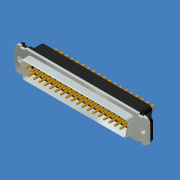
# Autodesk Inventor part: DBConnector
Saved by Autodesk Inventor 2019 (Build 230136000, 136)
## iProperties
Shininess: 64.0
Angle Display Precision: 2
Document Length Units: 11272
Document Angle Units: 11279
Document Time Units: 11290
Document Mass Units: 11286
Document Length Units Precision: 3
Document Angle Units Precision: 2
Compacted: True
Created: 2001-12-01
Part Number: DBConnector
Description: Dsub 37 Pin, 2 Row, Male
Document SubType Name: Modeling
Designer: Charles Bliss
Material: Generic
Density: 1 g/cm^3
Appearance: Zinc
Categories: <MemberInstance><Categories><Category DisplayName="" Mnemonic="CABLEANDHARNESS" InternalName="e4a7e005-5e42-4d16-b293-125e7f0d0512"><Category DisplayName="" Mnemonic="CONNECTORS" InternalName="6f634eba-a678-4820-a31d-2c2d5ee6728e"><CategoryParameter DisplayName="" Mnemonic="REFDES" InternalName="c3740e8c-60ab-4d5d-8584-52b73222f2f0"/><Category DisplayName="" Mnemonic="RIBBONCABLE" InternalName="27621a3d-53ec-49ed-8225-e2ac65e8eb52"/></Category></Category></Categories><FamilyTemplate><FamilyTemplateParameters></FamilyTemplateParameters></FamilyTemplate><CategoryParameterMap><ParamToTemplateMap><ParamToTemplate CategoryParameter="//CategoryParameter[@InternalName='c3740e8c-60ab-4d5d-8584-52b73222f2f0']" ConstantValue=""/></ParamToTemplateMap></CategoryParameterMap></MemberInstance>
Density: 0.0
Volumn: 0.0
Area: 0.0
PropertySet Name: Model Information
Control State: 0
Master: False
Checked Out: False
Author: Charles Bliss
Autodesk Inventor part; units mm, degrees
ref_plane "YZ Plane" through (0, 0, 0) normal (1, 0, 0) x (0, 1, 0)
ref_plane "XZ Plane" through (0, 0, 0) normal (0, 1, 0) x (-1, 0, 0)
ref_plane "XY Plane" through (0, 0, 0) normal (0, 0, 1) x (1, 0, 0)
sketch "Sketch1" plane through (0, 0, 0) normal (0, 0, 1) x (1, 0, 0)
  line L0 (-29.3316, 6.2738) -> (29.3316, 6.2738)
  line L1 (29.3316, 6.2738) -> (29.3316, 5.4179)
  line L2 (29.3316, 5.4179) -> (31.75, 5.4179)
  line L3 (31.75, 5.4179) -> (31.75, 6.2738)
  line L4 (31.75, 6.2738) -> (32.2399, 6.2738)
  arc A0 (34.6583, 3.8554) -> (32.2399, 6.2738) centre (32.2399, 3.8554) ccw
  line L5 (-29.3316, 6.2738) -> (-29.3316, 5.4179)
  line L6 (-29.3316, 5.4179) -> (-31.75, 5.4179)
  line L7 (-31.75, 5.4179) -> (-31.75, 6.2738)
  line L8 (-31.75, 6.2738) -> (-32.2399, 6.2738)
  arc A1 (-32.2399, 6.2738) -> (-34.6583, 3.8554) centre (-32.2399, 3.8554) ccw
  line L9 (-34.6583, 0) -> (34.6583, 0) construction
  line L10 (-29.3316, -6.2738) -> (29.3316, -6.2738)
  line L11 (-29.3316, -6.2738) -> (-29.3316, -5.4179)
  line L12 (-29.3316, -5.4179) -> (-31.75, -5.4179)
  line L13 (-31.75, -5.4179) -> (-31.75, -6.2738)
  line L14 (-31.75, -6.2738) -> (-32.2399, -6.2738)
  arc A2 (-34.6583, -3.8554) -> (-32.2399, -6.2738) centre (-32.2399, -3.8554) ccw
  line L15 (29.3316, -6.2738) -> (29.3316, -5.4179)
  line L16 (29.3316, -5.4179) -> (31.75, -5.4179)
  line L17 (31.75, -5.4179) -> (31.75, -6.2738)
  line L18 (31.75, -6.2738) -> (32.2399, -6.2738)
  arc A3 (32.2399, -6.2738) -> (34.6583, -3.8554) centre (32.2399, -3.8554) ccw
  line L19 (-34.6583, 3.8554) -> (-34.6583, -3.8554)
  line L20 (34.6583, 3.8554) -> (34.6583, -3.8554)
  line L21 (-27.1708, -3.1583) -> (-28.0576, 1.8711)
  arc A4 (-25.802, 4.5593) -> (-28.0576, 1.8711) centre (-25.802, 2.2689) ccw
  line L22 (-25.802, 4.5593) -> (25.802, 4.5593)
  arc A5 (28.0576, 1.8711) -> (25.802, 4.5593) centre (25.802, 2.2689) ccw
  line L23 (28.0576, 1.8711) -> (27.1708, -3.1583)
  arc A6 (25.5011, -4.5593) -> (27.1708, -3.1583) centre (25.5011, -2.8639) ccw
  line L24 (25.5011, -4.5593) -> (-25.5011, -4.5593)
  arc A7 (-27.1708, -3.1583) -> (-25.5011, -4.5593) centre (-25.5011, -2.8639) ccw
  line L25 (0, 6.2738) -> (0, -6.2738) construction
  line L26 (0, 4.5593) -> (0, -4.5593) construction
  line L27 (-25.5011, -4.1783) -> (25.5011, -4.1783)
  arc A8 (25.5011, -4.1783) -> (26.7956, -3.0921) centre (25.5011, -2.8639) ccw
  line L28 (26.7956, -3.0921) -> (27.6824, 1.9373)
  arc A9 (27.6824, 1.9373) -> (25.802, 4.1783) centre (25.802, 2.2689) ccw
  line L29 (25.802, 4.1783) -> (-25.802, 4.1783)
  arc A10 (-25.802, 4.1783) -> (-27.6824, 1.9373) centre (-25.802, 2.2689) ccw
  line L30 (-27.6824, 1.9373) -> (-26.7956, -3.0921)
  arc A11 (-26.7956, -3.0921) -> (-25.5011, -4.1783) centre (-25.5011, -2.8639) ccw
  circle A12 centre (-31.75, 0) radius 1.524
  circle A13 centre (31.75, 0) radius 1.524
  line L31 (-31.75, 0) -> (0, 0) construction
  line L32 (0, 0) -> (31.75, 0) construction
  line L33 (27.7114, 6.2738) -> (27.7114, 2.2689) construction
  line L34 (-27.7114, 6.2738) -> (-27.7114, 2.2689) construction
  line L35 (-27.9785, 1.4224) -> (27.9785, 1.4224) construction
  line L36 (-27.4769, -1.4224) -> (27.4769, -1.4224) construction
  circle A14 centre (-25.146, 1.4224) radius 0.4953
  circle A15 centre (-23.749, -1.4224) radius 0.4953
  line L37 (-26.9753, -4.2672) -> (26.9753, -4.2672) construction
  circle A16 centre (-25.146, -4.2672) radius 0.4953
  point P0 (0, -1.4224)
  dimension "d0" = 10
  dimension "HoleCtr" = 63.5
  dimension "OAL" = 69.3166
  dimension "ShellLen" = 55.4228
  dimension "ShellWid" = 8.3566
  dimension "HoleDia" = 3.048
  dimension "d6" = 0.381
  dimension "d7" = 2.4184
  dimension "d8" = 0.8559
  dimension "d9" = 2.4184
  dimension "OAW" = 12.5476
  dimension "d11" = 1.3144
  dimension "PinVertDist" = 2.8448
  dimension "PinDia" = 0.9906
  dimension "Pin1Offset" = 25.146
  dimension "d19" = 1.397
  dimension "d34" = 1.9094
  dimension "CLoffset" = 2.7559
  dimension "d52" = 2.8448
  constraints: 76 end point, 26 point on circle, 17 centre point, 16 tangent, 14 point on line, 14 symmetric about line, 10 parallel, 8 midpoint, 6 equal length, 6 equal radius, 5 collinear, 4 perpendicular, 3 horizontal, 3 vertical alignment, 2 coincident, 2 vertical, 18 other
  measures "d0" angle of L21 L19
  measures "HoleCtr" diameter of A12.centre L25
  measures "OAL" distance between parallel lines of L20 L19
  measures "ShellLen" distance between parallel lines of L33 L34
  measures "ShellWid" distance between parallel lines of L27 L29
  measures "HoleDia" diameter of A13
  measures "d6" distance between parallel lines of L30 L21
  measures "d7" distance of L6.start L6.end
  measures "d8" distance of L0.start L6.start
  measures "d9" radius of A1
  measures "OAW" distance between parallel lines of L10 L0
  measures "d11" radius of A8
  measures "PinVertDist" distance between parallel lines of L36 L35
  measures "PinDia" diameter of A15
  measures "Pin1Offset" distance from line of A14.centre L26
  measures "d19" horizontal distance of A15.centre A14.centre
  measures "d34" radius of A10
  measures "CLoffset" distance between parallel lines of L27 L36
  measures "d52" distance between parallel lines of L37 L36
extrude "Extrusion1" add sketch "Sketch1" along normal blind 1.27 contours L0 L1 L2 L3 L4 A0 L20 A3 L18 L17 L16 L15 L10 L11 L12 L13 L14 A2 L19 A1 L8 L7 L6 L5 | L21 A4 L22 A5 L23 A6 L24 A16 L27 A8 L28 A9 L29 A10 L30 A11 A7 | A16 A11 L27 L24 A7 | A7 L24 A16
extrude "Extrusion2" add sketch "Sketch1" along normal blind 5.08 contours L21 A4 L22 A5 L23 A6 L24 A16 L27 A8 L28 A9 L29 A10 L30 A11 A7 | A16 A11 L27 L24 A7
fillet "Fillet4" radius 0.381 8 edges at (-26.5909, -4.1626, 5.08) (-27.6142, -0.6436, 5.08) (-27.5565, 3.7411, 5.08) (0, 4.5593, 5.08) (27.5565, 3.7411, 5.08) (27.6142, -0.6436, 5.08) (26.5909, -4.1626, 5.08) (0, -4.5593, 5.08)
extrude "Pin1" add sketch "Sketch1" along normal blind 5.08 contours A14
extrude "Pin2" add sketch "Sketch1" along normal blind 5.08 contours A15
extrude "Pin50" [suppressed]
fillet "Fillet1" radius 0.4953 1 edges at (-25.6413, 1.4224, 5.08)
fillet "Fillet2" radius 0.4953 1 edges at (-24.2443, -1.4224, 5.08)
fillet "Fillet50" [suppressed]
sketch "Sketch2" plane through (0, 0, 0) normal (0, 0, -1) x (-1, 0, 0)
  circle A0 centre (-31.75, 0) radius 1.524 projected
  circle A1 centre (31.75, 0) radius 1.524 projected
  line L0 (29.3316, 6.2738) -> (-29.3316, 6.2738) projected
  line L1 (-29.3316, 6.2738) -> (-29.3316, 5.4179) projected
  line L2 (-29.3316, 5.4179) -> (-31.75, 5.4179) projected
  line L3 (-31.75, 5.4179) -> (-31.75, 6.2738) projected
  line L4 (-31.75, 6.2738) -> (-32.2399, 6.2738) projected
  arc A2 (-32.2399, 6.2738) -> (-34.6583, 3.8554) centre (-32.2399, 3.8554) ccw projected
  line L5 (-34.6583, 3.8554) -> (-34.6583, -3.8554) projected
  arc A3 (-34.6583, -3.8554) -> (-32.2399, -6.2738) centre (-32.2399, -3.8554) ccw projected
  line L6 (-32.2399, -6.2738) -> (-31.75, -6.2738) projected
  line L7 (-31.75, -6.2738) -> (-31.75, -5.4179) projected
  line L8 (-31.75, -5.4179) -> (-29.3316, -5.4179) projected
  line L9 (-29.3316, -5.4179) -> (-29.3316, -6.2738) projected
  line L10 (-29.3316, -6.2738) -> (29.3316, -6.2738) projected
  line L11 (29.3316, -6.2738) -> (29.3316, -5.4179) projected
  line L12 (29.3316, -5.4179) -> (31.75, -5.4179) projected
  line L13 (31.75, -5.4179) -> (31.75, -6.2738) projected
  line L14 (31.75, -6.2738) -> (32.2399, -6.2738) projected
  arc A4 (32.2399, -6.2738) -> (34.6583, -3.8554) centre (32.2399, -3.8554) ccw projected
  line L15 (34.6583, -3.8554) -> (34.6583, 3.8554) projected
  arc A5 (34.6583, 3.8554) -> (32.2399, 6.2738) centre (32.2399, 3.8554) ccw projected
  line L16 (32.2399, 6.2738) -> (31.75, 6.2738) projected
  line L17 (31.75, 6.2738) -> (31.75, 5.4179) projected
  line L18 (31.75, 5.4179) -> (29.3316, 5.4179) projected
  line L19 (29.3316, 5.4179) -> (29.3316, 6.2738) projected
  line L20 (-29.0776, 6.0198) -> (29.0776, 6.0198)
  line L21 (29.0776, 6.0198) -> (29.0776, 5.1639)
  line L22 (29.0776, 5.1639) -> (32.004, 5.1639)
  line L23 (32.004, 5.1639) -> (32.004, 6.0198)
  line L24 (32.004, 6.0198) -> (32.2399, 6.0198)
  arc A6 (34.4043, 3.8554) -> (32.2399, 6.0198) centre (32.2399, 3.8554) ccw
  line L25 (34.4043, 3.8554) -> (34.4043, -3.8554)
  arc A7 (32.2399, -6.0198) -> (34.4043, -3.8554) centre (32.2399, -3.8554) ccw
  line L26 (32.2399, -6.0198) -> (32.004, -6.0198)
  line L27 (32.004, -6.0198) -> (32.004, -5.1639)
  line L28 (32.004, -5.1639) -> (29.0776, -5.1639)
  line L29 (29.0776, -5.1639) -> (29.0776, -6.0198)
  line L30 (29.0776, -6.0198) -> (-29.0776, -6.0198)
  line L31 (-29.0776, -6.0198) -> (-29.0776, -5.1639)
  line L32 (-29.0776, -5.1639) -> (-32.004, -5.1639)
  line L33 (-32.004, -5.1639) -> (-32.004, -6.0198)
  line L34 (-32.004, -6.0198) -> (-32.2399, -6.0198)
  arc A8 (-34.4043, -3.8554) -> (-32.2399, -6.0198) centre (-32.2399, -3.8554) ccw
  line L35 (-34.4043, -3.8554) -> (-34.4043, 3.8554)
  arc A9 (-32.2399, 6.0198) -> (-34.4043, 3.8554) centre (-32.2399, 3.8554) ccw
  line L36 (-32.2399, 6.0198) -> (-32.004, 6.0198)
  line L37 (-32.004, 6.0198) -> (-32.004, 5.1639)
  line L38 (-32.004, 5.1639) -> (-29.0776, 5.1639)
  line L39 (-29.0776, 5.1639) -> (-29.0776, 6.0198)
  dimension "d35" = 0.254
  constraints: 40 end point, 8 point on circle, 4 centre point, 23 other
  measures "d35" distance between parallel lines of L5 L35
extrude "Extrusion5" add sketch "Sketch2" along normal blind 1.6002 contours L20 L21 L22 L23 L24 A6 L25 A7 L26 L27 L28 L29 L30 L31 L32 L33 L34 A8 L35 A9 L36 L37 L38 L39
sketch "Sketch3" plane through (0, 0, -1.6002) normal (0, 0, -1) x (-1, 0, 0)
  line L0 (-27.101, 5.4483) -> (27.101, 5.4483)
  arc A0 (28.9814, 3.2073) -> (27.101, 5.4483) centre (27.101, 3.5389) ccw
  line L1 (28.9814, 3.2073) -> (27.7334, -3.8704)
  arc A1 (25.853, -5.4483) -> (27.7334, -3.8704) centre (25.853, -3.5389) ccw
  line L2 (25.853, -5.4483) -> (-25.853, -5.4483)
  arc A2 (-27.7334, -3.8704) -> (-25.853, -5.4483) centre (-25.853, -3.5389) ccw
  line L3 (-27.7334, -3.8704) -> (-28.9814, 3.2073)
  arc A3 (-27.101, 5.4483) -> (-28.9814, 3.2073) centre (-27.101, 3.5389) ccw
  line L4 (0, 0) -> (0, 5.4483) construction
  line L5 (0, 0) -> (0, -5.4483) construction
  line L6 (-29.0776, 6.0198) -> (29.0776, 6.0198) projected
  line L7 (-28.0576, 1.8711) -> (-27.1708, -3.1583) projected
  dimension "d86" = 1.9094
  dimension "d87" = 10.8966
  dimension "d88" = 57.9628
  constraints: 12 end point, 8 point on circle, 8 tangent, 4 centre point, 2 equal length, 2 horizontal alignment, 2 midpoint, 2 vertical, 1 equal radius, 1 parallel, 1 perpendicular
  measures "d86" radius of A2
  measures "d87" distance of L5.end L4.end
  measures "d88" distance of L1.start L3.end
extrude "Extrusion6" add sketch "Sketch3" along normal blind 5.08
sketch "Sketch4" plane through (0, 0, -6.6802) normal (0, 0, -1) x (-1, 0, 0)
  line L0 (23.241, -0.9144) -> (24.257, -0.9144)
  line L1 (24.257, -0.9144) -> (24.257, -1.9304)
  line L2 (24.257, -1.9304) -> (23.241, -1.9304)
  line L3 (23.241, -1.9304) -> (23.241, -0.9144)
  line L4 (24.638, 1.9304) -> (25.654, 1.9304)
  line L5 (25.654, 1.9304) -> (25.654, 0.9144)
  line L6 (25.654, 0.9144) -> (24.638, 0.9144)
  line L7 (24.638, 0.9144) -> (24.638, 1.9304)
  line L8 (25.654, -4.7752) -> (24.638, -4.7752)
  line L9 (24.638, -4.7752) -> (24.638, -3.7592)
  line L10 (24.638, -3.7592) -> (25.654, -3.7592)
  line L11 (25.654, -3.7592) -> (25.654, -4.7752)
  point P0 (25.146, 1.4224)
  point P1 (23.749, -1.4224)
  point P2 (23.749, -1.4224)
  point P3 (25.146, 1.4224)
  point P4 (25.146, -4.2672)
  point P5 (25.146, -4.2672)
  dimension "d46" = 1.016
  constraints: 24 end point, 3 coincident, 3 horizontal, 2 parallel, 21 other
  measures "d46" distance of L4.end L5.end
extrude "Extrusion7" add sketch "Sketch4" along normal blind 5.08 contours L0 L1 L2 L3
extrude "Extrusion8" add sketch "Sketch4" along normal blind 5.08 contours L4 L5 L6 L7
extrude "ExtrudeSgr50" [suppressed]
chamfer "Chamfer1" distance 0.3048 angle 45 4 edges at (-25.146, 0.9144, -11.7602) (-24.638, 1.4224, -11.7602) (-25.146, 1.9304, -11.7602) (-25.654, 1.4224, -11.7602)
chamfer "Chamfer2" distance 0.3048 angle 45 4 edges at (-23.241, -1.4224, -11.7602) (-23.749, -0.9144, -11.7602) (-24.257, -1.4224, -11.7602) (-23.749, -1.9304, -11.7602)
chamfer "Chamfer50" [suppressed]
pattern_linear "Pattern1" count 19 spacing 2.794 along (1, 0, 0) of "Pin1", "Extrusion8", "Fillet1", "Chamfer1"
pattern_linear "Pattern2" count 18 spacing 2.794 along (1, 0, 0) of "Pin2", "Extrusion7", "Fillet2", "Chamfer2"
pattern_linear "Pattern50" [suppressed]
pattern_linear "Pattern15" [suppressed]
extrude "Female" [suppressed]
extrude "Socket1" [suppressed]
extrude "Socket2" [suppressed]
extrude "Socket50" [suppressed]
pattern_linear "Pattern5" [suppressed]
pattern_linear "Pattern6" [suppressed]
pattern_linear "Pattern7" [suppressed]
equation "\"d19\" = 0.5 * PinSpace"
equation "\"d52\" = PinVertDist"
equation "\"d63\" = d6"
equation "\"d26\" = d24"
equation "\"d53\" = d24"
equation "\"d44\" = 0.5 * PinDia"
equation "\"d45\" = 0.5 * PinDia"
equation "\"d55\" = 0.5 * PinDia"
equation "\"d56\" = d24"
equation "\"d47\" = 0.3 * d46"
equation "\"d48\" = 0.3 * d46"
equation "\"d49\" = 0.3 * d46"
equation "\"d50\" = 0.3 * d46"
equation "\"d58\" = 0.2 * d46"
equation "\"d59\" = 0.2 * d46"
equation "\"d66\" = PinSpace"
equation "\"d30\" = PinSpace"
equation "\"d33\" = PinSpace"
equation "\"d62\" = PinSpace"
equation "\"d77\" = PinSpace"
equation "\"d80\" = PinSpace"
equation "\"d83\" = PinSpace"
equation "\"PinSpace\" = 2.794"
equation "\"RowOffset\" = 1.397"
equation "\"d24\" = 5.08"
body "Solid1"
